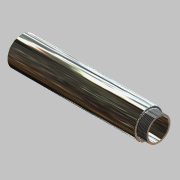
# Autodesk Inventor part: YTP-AP-E09-R1.0
Saved by Autodesk Inventor 2020.4 (Build 244396010, 396A)
## iProperties
RuleStatus: InUse
AfterDocNew0: iPropertyEnforcement
BeforeDocSave0: Materialprüfung
Created: 2021-08-29
Part Number: YTP-AP-E09-R1.0
Material: Allgemein
Document SubType Name: Modeling
Designer: Uwe Wieser
Mass: 3.13045 g
Surface Area: 38.3381 cm^2
Volume: 3.13045 cm^3
Density: 1 g/cm^3
Appearance: Chrom - poliert
Project: Airbrush
Description: Endkappe
Werkstoff: 1.4301
Author: Uwe Wieser
Autodesk Inventor part; units mm, degrees
ref_plane "YZ Plane" through (0, 0, 0) normal (1, 0, 0) x (0, 1, 0)
ref_plane "XZ Plane" through (0, 0, 0) normal (0, 1, 0) x (-1, 0, 0)
ref_plane "XY Plane" through (0, 0, 0) normal (0, 0, 1) x (1, 0, 0)
sketch "Skizze1" plane through (0, 0, 0) normal (0, 0, 1) x (1, 0, 0)
  line L0 (0, 5) -> (-3.8, 5)
  line L1 (-55.8, 4.25) -> (0, 4.25)
  line L2 (-4, 5.8) -> (-4, 5.2)
  line L3 (-4.2, 6) -> (-56.8, 6)
  line L4 (-57, 5.8) -> (-57, 4.25)
  line L5 (-68.4497, 0) -> (11.4083, 0) projected
  line L6 (0, -1.2083) -> (0, 7.2497) projected
  line L7 (0, 5) -> (0, 4.25)
  arc A0 (-4, 5.2) -> (-3.8, 5) centre (-3.8, 5.2) ccw
  arc A1 (-56.8, 6) -> (-57, 5.8) centre (-56.8, 5.8) ccw
  line L8 (-57, 4.25) -> (-57, 0)
  line L9 (-57, 0) -> (-56, 0)
  line L10 (-56, 4.05) -> (-56, 0)
  arc A2 (-55.8, 4.25) -> (-56, 4.05) centre (-55.8, 4.05) ccw
  arc A3 (-4, 5.8) -> (-4.2, 6) centre (-4.2, 5.8) ccw
  point P0 (-4, 6)
  dimension "d0" = 8.5
  dimension "d1" = 10
  dimension "d2" = 12
  dimension "d3" = 4
  dimension "d4" = 57
  dimension "d5" = 0.2
  dimension "d9" = 1
  dimension "d10" = 0.2
  dimension "d11" = 0.2
  constraints: 18 end point, 8 point on circle, 8 tangent, 5 point on line, 4 centre point, 2 perpendicular, 1 collinear, 1 equal radius, 1 horizontal, 1 vertical
  measures "d0" diameter of L1 L5
  measures "d1" diameter of L0 L5
  measures "d2" diameter of L3 L5
  measures "d3" distance between parallel lines of L6 L2
  measures "d4" distance between parallel lines of L6 L4
  measures "d5" radius of A0
  measures "d9" distance between parallel lines of L8 L10
  measures "d10" radius of A2
  measures "d11" radius of A3
revolve "Umdrehung1" add sketch "Skizze1" angle 360 about axis through (-10, 0, 0) along (1, 0, 0) contours L6 L1 A2 L10 L5 L8 L4 A1 L3 A3 L2 A0 L0
thread "Gewinde1" size "M10x0.5" class "6g" standard "ISO Metric profile" full length
